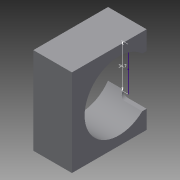
# Autodesk Inventor part: Noke_holder
Saved by Autodesk Inventor 2015 SP2 (Build 190223200, 223)
## iProperties
Created: 2016-08-30
Part Number: Noke_holder
Material: Generic
Document SubType Name: Modeling
Designer: jm799
Density: 1 g/cm^3
Appearance: Default
Author: jm799
Autodesk Inventor part; units mm, degrees
ref_plane "YZ Plane" through (0, 0, 0) normal (1, 0, 0) x (0, 1, 0)
ref_plane "XZ Plane" through (0, 0, 0) normal (0, 1, 0) x (-1, 0, 0)
ref_plane "XY Plane" through (0, 0, 0) normal (0, 0, 1) x (1, 0, 0)
sketch "Sketch1" plane through (0, 0, 0) normal (0, 1, 0) x (-1, 0, 0)
  line L0 (16.2222, 35.2121) -> (-14.7778, 35.2121)
  line L1 (-14.7778, 35.2121) -> (-14.7778, -34.7879)
  line L2 (-14.7778, -34.7879) -> (16.2222, -34.7879)
  line L3 (16.2222, -34.7879) -> (16.2222, 35.2121)
  point P0 (0, 0)
  dimension "d0" = 70
  dimension "d1" = 31
  constraints: 8 end point, 2 parallel, 1 horizontal, 1 perpendicular
  measures "d0" distance of L0.end L1.end
  measures "d1" distance of L0.start L0.end
extrude "Extrusion1" add sketch "Sketch1" along normal blind 60
sketch "Sketch2" plane through (0, 60, 0) normal (0, 1, 0) x (1, 0, 0)
  line L0 (0, -17.35) -> (0, 17.35)
  point P0 (0, 0)
  point P1 (0, 0)
  dimension "d4" = 34.7
  constraints: 2 end point, 1 coincident, 1 midpoint, 1 vertical
  measures "d4" distance of L0.start L0.end
sketch "Sketch3" plane through (14.7778, 0, 35.2121) normal (1, 0, 0) x (0, 0, -1)
  circle A0 centre (35.2121, 37.6844) radius 27.5
  point P0 (35.2121, 0)
  dimension "d5" = 55
  constraints: 1 centre point
  measures "d5" diameter of A0
hole "Hole1" at (14.7778, 37.6844, 0) direction (-1, 0, 0) diameter 55 end through all
sketch "Sketch4" plane through (0, 60, 0) normal (0, 1, 0) x (1, 0, 0)
  line L0 (14.7778, -16.0705) -> (-16.2222, -16.0705) projected
  circle A0 centre (0, -16.0705) radius 4
  point P0 (0, 0)
  dimension "d13" = 8
  constraints: 1 centre point, 1 point on line
  measures "d13" diameter of A0
sketch "Sketch5" plane through (0, 60, 0) normal (0, 1, 0) x (1, 0, 0)
  line L0 (-16.2222, 16.0705) -> (14.7778, 16.0705) projected
  circle A0 centre (0, 16.0705) radius 4
  point P0 (0, 0)
  dimension "d14" = 8
  constraints: 1 centre point, 1 point on line
  measures "d14" diameter of A0
hole "Hole2" at (0, 60, 16.0705) direction (0, -1, 0) diameter 8 depth 8 tip angle 118
hole "Hole3" at (0, 60, -16.0705) direction (0, -1, 0) diameter 8 depth 8 tip angle 118
sketch "Sketch6" plane through (0, 60, 0) normal (0, 1, 0) x (1, 0, 0)
  arc A0 (-4, -16.0705) -> (4, -16.0705) centre (0, -16.0705) ccw projected
  line L0 (0, -20.0705) -> (14.7778, -20.0705)
  line L1 (14.7778, -20.0705) -> (14.7778, -16.0705)
  line L2 (14.7778, -16.0705) -> (0, -16.0705)
  line L3 (14.7778, -16.0705) -> (4, -16.0705) projected
  line L4 (0, -16.0705) -> (0, -20.0705)
  point P0 (0, 0)
  constraints: 8 end point, 1 collinear, 1 horizontal, 1 perpendicular, 1 point on circle, 1 tangent, 1 vertical
extrude "Extrusion2" cut sketch "Sketch6" against normal blind 10 contours A0 L2 L1 L0
sketch "Sketch7" plane through (0, 60, 0) normal (0, 1, 0) x (1, 0, 0)
  arc A0 (4, 16.0705) -> (-4, 16.0705) centre (0, 16.0705) ccw projected
  line L0 (0, 20.0705) -> (14.7778, 20.0705)
  line L1 (14.7778, 16.0705) -> (14.7778, 34.7879) projected
  line L2 (14.7778, 20.0705) -> (14.7778, 16.0705)
  line L3 (14.7778, 16.0705) -> (0, 16.0705)
  line L4 (0, 16.0705) -> (0, 20.0705)
  point P0 (0, 0)
  constraints: 8 end point, 2 horizontal, 1 perpendicular, 1 point on circle, 1 point on line, 1 tangent, 1 vertical
extrude "Extrusion3" cut sketch "Sketch7" against normal blind 10
body "Solid1"
